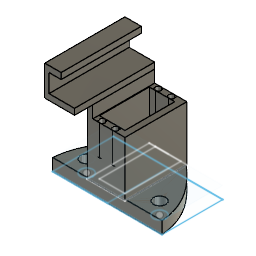
servo holer (Autodesk Fusion 360 design; units mm, degrees)
part number: 2026-03-11-01-15-29-586
part number: 2026-03-11-04-13-13-850
Autodesk Fusion 360 part; units mm, degrees
note: some values were not read from the file. Chosen so that the rebuilt part matches the saved one: which bodies a step acts on. Set by a fixed rule: which sketch regions a step uses.
sketch "Sketch1" plane through (0, 0, 0) normal (0, 0, 1) x (1, 0, 0)
  line L0 (15, 0) -> (105, 0)
  line L1 (105, 50) -> (15, 50)
  circle A0 centre (30, 13) radius 5
  circle A1 centre (90, 13) radius 5
  line L2 (60, 0) -> (15, 0)
  line L3 (15, 0) -> (105, 0)
  line L4 (105, 0) -> (105, 50)
  line L5 (105, 50) -> (15, 50)
  line L6 (15, 50) -> (15, 0)
  line L7 (60, 50) -> (60, 0)
  dimension "d3" = 10
  dimension "d6" = 50
  dimension "d56" = 13
  dimension "d57" = 13
  constraint horizontal L0
  constraint horizontal L1
  constraint horizontal L3
  constraint vertical L4
  constraint horizontal L5
  constraint vertical L6
  constraint coincident L0 L2.start
  constraint midpoint L5 L7.start
  measures "d3" diameter of A0
  measures "d6" distance of L0.start L1.end
  measures "d56" distance of A0.centre L2
  measures "d57" distance of L0 A1.centre
extrude "Extrude1" add sketch "Sketch1" along normal blind 10 makes body 1
sketch "Sketch2" plane through (0, 0, 10) normal (0, 0, 1) x (-1, 0, 0)
  circle A0 centre (-30, -13) radius 5
  circle A1 centre (-90, -13) radius 5
  line L0 (-15, -50) -> (-15, 0)
  line L1 (-15, 0) -> (-105, 0)
  line L2 (-105, 0) -> (-105, -50)
  line L3 (-105, -50) -> (-15, -50)
  line L4 (-60, -50) -> (-49.5, -50)
  line L5 (-49.5, -50) -> (-70.5, -50)
  line L6 (-70.5, -50) -> (-70.5, -4)
  line L7 (-70.5, -4) -> (-49.5, -4)
  line L8 (-49.5, -4) -> (-49.5, -50)
  line L9 (-49.5, -50) -> (-44.5, -50)
  line L10 (-44.5, -50) -> (-75.5, -50)
  line L11 (-75.5, -50) -> (-75.5, 1)
  line L12 (-75.5, 1) -> (-44.5, 1)
  line L13 (-44.5, 1) -> (-44.5, -50)
  dimension "d7" = 10.5
  dimension "d8" = 21
  dimension "d9" = 46
  dimension "d10" = 5
  dimension "d11" = 31
  dimension "d12" = 51
  constraint midpoint L3 L4.start
  constraint parallel L3 L4
  constraint horizontal L5
  constraint vertical L6
  constraint horizontal L7
  constraint vertical L8
  constraint perpendicular L8 L9
  constraint horizontal L10
  constraint vertical L11
  constraint horizontal L12
  constraint vertical L13
  measures "d7" distance of L4.start L4.end
  measures "d8" distance of L4.end L5.end
  measures "d9" distance of L4.end L7.end
  measures "d10" distance of L4.end L9.end
  measures "d11" distance of L9.end L10.end
  measures "d12" distance of L9.end L12.end
extrude "Extrude2" add sketch "Sketch2" along normal blind 15 contours L3 L4 L5 L6 L7 L8 L10 bodies 1
extrude "Extrude3" add sketch "Sketch2" along normal blind 45 contours L1 L3 L6 L7 L8 L9 L10 L11 L13 | L1 L11 L12 L13 bodies 1
sketch "Sketch3" plane through (0, 50, 0) normal (0, 1, 0) x (-1, 0, 0)
  line L0 (-105, 0) -> (-15, 0)
  line L1 (-15, 0) -> (-15, 10)
  line L2 (-15, 10) -> (-44.5, 10)
  line L3 (-44.5, 10) -> (-44.5, 55)
  line L4 (-44.5, 55) -> (-49.5, 55)
  line L5 (-49.5, 55) -> (-49.5, 25)
  line L6 (-49.5, 25) -> (-70.5, 25)
  line L7 (-70.5, 25) -> (-70.5, 55)
  line L8 (-70.5, 55) -> (-75.5, 55)
  line L9 (-75.5, 55) -> (-75.5, 10)
  line L10 (-75.5, 10) -> (-105, 10)
  line L11 (-105, 10) -> (-105, 0)
  line L12 (-49.5, 25) -> (-49.5, 35)
  line L13 (-49.5, 35) -> (-70.5, 35)
  line L14 (-70.5, 35) -> (-70.5, 55)
  line L15 (-70.5, 55) -> (-49.5, 55)
  line L16 (-49.5, 55) -> (-49.5, 35)
  constraint coincident L5.end L6.start
  constraint coincident L5 L12.end
  constraint horizontal L13
  constraint vertical L14
  constraint horizontal L15
  constraint vertical L16
  constraint coincident L7.end L8.start
extrude "Extrude4" add sketch "Sketch3" against normal blind 5 contours L5 L7 L13 L14 L15 L16 bodies 1
sketch "Sketch4" plane through (0, 0, 55) normal (0, 0, 1) x (-1, 0, 0)
  line L0 (-70.5, -45) -> (-70.5, -4)
  line L1 (-70.5, -4) -> (-49.5, -4)
  line L2 (-49.5, -4) -> (-49.5, -45)
  line L3 (-49.5, -45) -> (-70.5, -45)
  line L4 (-75.5, -50) -> (-44.5, -50)
  line L5 (-44.5, -50) -> (-44.5, 1)
  line L6 (-44.5, 1) -> (-75.5, 1)
  line L7 (-75.5, 1) -> (-75.5, -50)
  line L8 (-70.5, -45) -> (-65.5, -45)
  line L9 (-65.5, -45) -> (-65.5, -50)
  circle A0 centre (-65.5, -47.5) radius 2.5
  line L10 (-75.5, -24.5) -> (-70.5, -24.5)
  line L11 (-60, -45) -> (-60, -50)
  circle A1 centre (-54.5, -47.5) radius 2.5
  circle A2 centre (-65.5, -1.5) radius 2.5
  circle A3 centre (-54.5, -1.5) radius 2.5
  dimension "d19" = 5
  dimension "d20" = 5
  constraint coincident L0.start L3.end
  constraint perpendicular L0 L8
  constraint perpendicular L8 L9
  constraint midpoint L9 A0.centre
  constraint midpoint L7 L10.start
  constraint midpoint L0 L10.end
  constraint midpoint L3 L11.start
  constraint midpoint L4 L11.end
  constraint symmetric A0 L11 A1
  constraint symmetric A0 L10 A2
  constraint symmetric L10 A1 A3
  measures "d19" distance of L0.start L8.end
  measures "d20" diameter of A0
extrude "Extrude5" cut sketch "Sketch4" against normal blind 25 contours L9 A0 | L9 A0 | A2 | A1 | A3 bodies 1
sketch "Sketch5" plane through (0, 0, 55) normal (0, 0, 1) x (-1, 0, 0)
  arc A0 (-54.5, -50) -> (-54.5, -45) centre (-54.5, -47.5) ccw
  line L0 (-54.5, -50) -> (-44.5, -50)
  line L1 (-44.5, -50) -> (-44.5, 1)
  line L2 (-44.5, 1) -> (-54.5, 1)
  arc A1 (-54.5, -4) -> (-54.5, 1) centre (-54.5, -1.5) ccw
  line L3 (-54.5, -4) -> (-49.5, -4)
  line L4 (-49.5, -4) -> (-49.5, -45)
  line L5 (-49.5, -45) -> (-54.5, -45)
  line L6 (-44.5, -50) -> (-49, -50)
  line L7 (-49, -50) -> (-49, 1)
  line L8 (-49, 1) -> (-44.5, 1)
  line L9 (-44.5, 1) -> (-44.5, -50)
  constraint horizontal L6
  constraint vertical L7
  constraint horizontal L8
  constraint vertical L9
  constraint coincident L2 L7.end
  constraint coincident L0.end L1.start
extrude "Extrude6" add sketch "Sketch5" along normal blind 15 contours L0 L1 L2 L6 L7 L8 L9 bodies 1
sketch "Sketch6" plane through (0, 0, 10) normal (0, 0, 1) x (-1, 0, 0)
  spline S0 degree 5 poles (-105, 0) (-104.9095, -1.0615) (-104.6822, -3.1788) (-104.2027, -6.3381) (-103.2817, -10.5165) (-101.6307, -15.6792) (-99.4414, -20.777) (-96.6795, -25.8057) (-93.3439, -30.7653) (-89.4733, -35.6602) (-85.1155, -40.4964) (-81.2751, -44.3227) (-78.2087, -47.1699) (-76.0831, -49.0583) (-75, -50) knots 0 0 0 0 0 0 0.1 0.2 0.3 0.4 0.5 0.6 0.7 0.8 0.9 1 1 1 1 1 1
  line L0 (-60, -50) -> (-60, 0)
  spline S1 degree 5 poles (-15, 0) (-15.0905, -1.0615) (-15.3178, -3.1788) (-15.7973, -6.3381) (-16.7183, -10.5165) (-18.3693, -15.6792) (-20.5586, -20.777) (-23.3205, -25.8057) (-26.6561, -30.7653) (-30.5267, -35.6602) (-34.8845, -40.4964) (-38.7249, -44.3227) (-41.7913, -47.1699) (-43.9169, -49.0583) (-45, -50) knots 0 0 0 0 0 0 0.1 0.2 0.3 0.4 0.5 0.6 0.7 0.8 0.9 1 1 1 1 1 1
  line L1 (-105.5396, 6.3257) -> (-104.4604, -6.3257)
  line L2 (-80.4688, -45.2452) -> (-69.5312, -54.7548)
  line L3 (-14.4604, 6.3257) -> (-15.5396, -6.3257)
  line L4 (-39.5312, -45.2452) -> (-50.4688, -54.7548)
  line L5 (-105, 0) -> (-105, -50)
  line L6 (-105, -50) -> (-75, -50)
  line L7 (-15, 0) -> (-15, -50)
  line L8 (-15, -50) -> (-45, -50)
  point P0 (-97.707, -23.7902)
  point P1 (-22.293, -23.7902)
  constraint midpoint S0.start L1
  constraint midpoint S0.end L2
  constraint symmetric S0.start L0 S1.start
  constraint symmetric P0 L0 P1
  constraint symmetric S0.end L0 S1.end
  constraint symmetric L0 L1.start L3.start
  constraint symmetric L0 L1.end L3.end
  constraint symmetric L0 L2.start L4.start
  constraint symmetric L0 L2.end L4.end
  constraint vertical L5
  constraint perpendicular L5 L6
  constraint perpendicular L6 L7
extrude "Extrude7" cut sketch "Sketch6" against normal blind 15 bodies 1
sketch "Sketch7" plane through (44.5, 0, 0) normal (-1, 0, 0) x (0, -1, 0)
  line L0 (0, 10) -> (1, 10)
  line L1 (1, 10) -> (1, 70)
  line L2 (1, 70) -> (-50, 70)
  line L3 (-50, 70) -> (-50, 10)
  line L4 (-50, 10) -> (-49.5635, 10)
  line L5 (-49.5635, 10) -> (0, 10)
  line L6 (-50, 70) -> (1, 70)
  line L7 (1, 70) -> (1, 65)
  line L8 (1, 65) -> (-50, 65)
  line L9 (-50, 65) -> (-50, 70)
  dimension "d35" = 5
  constraint horizontal L6
  constraint vertical L7
  constraint horizontal L8
  constraint vertical L9
  constraint coincident L2.end L3.start
  measures "d35" distance of L2.end L8.end
extrude "Extrude8" add sketch "Sketch7" along normal blind 20 contours L1 L2 L3 L6 L7 L8 L9 bodies 1
sketch "Sketch8" plane through (0, 0, 70) normal (0, 0, 1) x (-1, 0, 0)
  line L0 (-24.5, 1) -> (-49, 1)
  line L1 (-49, 1) -> (-49, -50)
  line L2 (-49, -50) -> (-24.5, -50)
  line L3 (-24.5, -50) -> (-24.5, 1)
  line L4 (-24.5, -50) -> (-29, -50)
  line L5 (-29, -50) -> (-29, 1)
  line L6 (-29, 1) -> (-24.5, 1)
  line L7 (-24.5, 1) -> (-24.5, -50)
  constraint horizontal L4
  constraint vertical L5
  constraint horizontal L6
  constraint vertical L7
  constraint coincident L0 L5.end
  constraint coincident L2.end L3.start
extrude "Extrude9" add sketch "Sketch8" along normal blind 20 contours L0 L2 L3 L4 L5 L6 L7 bodies 1
sketch "Sketch9" plane through (29, 0, 0) normal (1, 0, 0) x (0, 1, 0)
  line L0 (-1, 70) -> (50, 70)
  line L1 (50, 70) -> (50, 90)
  line L2 (50, 90) -> (-1, 90)
  line L3 (-1, 90) -> (-1, 70)
  line L4 (-1, 90) -> (50, 90)
  line L5 (50, 90) -> (50, 84)
  line L6 (50, 84) -> (-1, 84)
  line L7 (-1, 84) -> (-1, 90)
  dimension "d40" = 51
  dimension "d41" = 6
  constraint horizontal L4
  constraint vertical L5
  constraint horizontal L6
  constraint vertical L7
  constraint coincident L2.end L3.start
  measures "d40" distance of L2.end L1.end
  measures "d41" distance of L2.end L6.end
extrude "Extrude10" add sketch "Sketch9" along normal blind 15 contours L1 L2 L3 L4 L5 L6 L7 bodies 1
extrude "Extrude11" cut 1 faces at (44, 16, 88) along direction (-1, 0, 0) blind 16 on bodies 1 bodies 1
extrude "Extrude12" cut 1 faces at (29, 33, 74.6667) along direction (-1, 0, 0) blind 1 on bodies 1 bodies 1
sketch "Sketch10" plane through (28, 0, 0) normal (1, 0, 0) x (0, 1, 0)
  line L0 (50, 70) -> (50, 90)
  line L1 (50, 90) -> (-1, 90)
  line L2 (-1, 90) -> (-1, 70)
  line L3 (-1, 70) -> (50, 70)
  line L4 (-1, 90) -> (50, 90)
  line L5 (50, 90) -> (50, 85)
  line L6 (50, 85) -> (-1, 85)
  line L7 (-1, 85) -> (-1, 90)
  constraint horizontal L4
  constraint vertical L5
  constraint horizontal L6
  constraint vertical L7
  constraint coincident L0 L5.end
  constraint coincident L1.end L2.start
extrude "Extrude13" add sketch "Sketch10" along normal blind 20 contours L0 L1 L2 L4 L5 L6 L7 bodies 1
sketch "Sketch11" plane through (0, -1, 0) normal (0, -1, 0) x (1, 0, 0)
  line L0 (49, 70) -> (28, 70)
  line L1 (28, 70) -> (28, 85)
  line L2 (28, 85) -> (48, 85)
  line L3 (48, 85) -> (48, 90)
  line L4 (48, 90) -> (24.5, 90)
  line L5 (24.5, 90) -> (24.5, 65)
  line L6 (24.5, 65) -> (44.5, 65)
  line L7 (44.5, 65) -> (44.5, 10)
  line L8 (44.5, 10) -> (75.5, 10)
  line L9 (75.5, 10) -> (75.5, 55)
  line L10 (75.5, 55) -> (65.5, 55)
  line L11 (65.5, 55) -> (54.5, 55)
  line L12 (54.5, 55) -> (49, 55)
  line L13 (49, 55) -> (49, 70)
  line L14 (44.5, 65) -> (49, 65)
  line L15 (65.5, 55) -> (65.5, 30)
  line L16 (65.5, 30) -> (65.5, 55)
  line L17 (54.5, 55) -> (54.5, 30)
  line L18 (54.5, 30) -> (54.5, 55)
  constraint coincident L6.end L7.start
  constraint coincident L13 L14.end
  constraint perpendicular L13 L14
extrude "Extrude14" add sketch "Sketch11" along normal blind 15 contours L0 L1 L2 L3 L4 L5 L6 L13 L14 bodies 1
extrude "Extrude15" cut 1 faces at (48, 28, 86.6667) along direction (-1, 0, 0) blind 10 on bodies 1 bodies 1
split "Split1" by plane through (44.5, -1, 65) normal (0, 0, -1) bodies 1 makes body 2 at (55, 26.7796, 0) makes body 2 at (58.1667, 50, 41.6667)
copy_body "Body->Comp2" bodies 2 removing the originals makes body 3 in component "Component"
component "Component" placed x (1, 0, 0) y (0, 1, 0) z (0, 0, 1) at (0, 0, 0)
